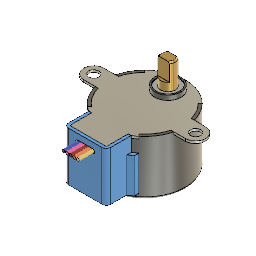
858 Stepper Motor 5VDC (Autodesk Fusion 360 design; units mm, degrees)
Autodesk Fusion 360 part; units mm, degrees
note: some values were not read from the file. Chosen so that the rebuilt part matches the saved one: which face or edge a step refers to.
sketch "base" plane through (0, 0, 0) normal (0, 0, 1) x (1, 0, 0)
  circle A0 centre (-17.5, 0) radius 1.75
  circle A1 centre (17.5, 0) radius 1.75
  line L0 (-17.5, 0) -> (17.5, 0) construction
  circle A2 centre (0, 0) radius 14
  line L1 (-21, 3.5) -> (21, 3.5)
  line L2 (21, 3.5) -> (21, -3.5)
  line L3 (21, -3.5) -> (-21, -3.5)
  line L4 (-21, -3.5) -> (-21, 3.5)
  line L5 (-7.3, -10.5) -> (7.3, -10.5)
  line L6 (7.3, -10.5) -> (7.3, -20.5)
  line L7 (7.3, -20.5) -> (-7.3, -20.5)
  line L8 (-7.3, -20.5) -> (-7.3, -10.5)
  line L9 (0, -10.5) -> (0, 0) construction
  circle A3 centre (0, 8) radius 4.5
  line L10 (0, 8) -> (0, 0) construction
  dimension "d1" = 3.5
  dimension "d2" = 3.5
  dimension "d5" = 7
  dimension "d6" = 3.5
  dimension "d7" = 3.5
  dimension "d9" = 3.5
  dimension "d10" = 28
  dimension "d12" = 10
  dimension "d14" = 17
  dimension "d15" = 14.6
  dimension "d16" = 9
  dimension "d17" = 8
  dimension "d56" = 35
  measures "d1" diameter of A0
  measures "d2" diameter of A1
  measures "d5" distance of L1.start L3.end
  measures "d6" distance of A2.centre L1
  measures "d7" distance of A1.centre L2
  measures "d9" distance of A0.centre L4
  measures "d10" diameter of A2
  measures "d12" distance of L5.start L7.end
  measures "d14" distance of L3 L7
  measures "d15" distance of L6.end L7.end
  measures "d16" diameter of A3
  measures "d17" distance of A2.centre A3.centre
  measures "d56" distance of A0.centre A1.centre
extrude "Extrude1" add sketch "base" against normal blind 0.8 contours A2 L1 L3 | A2 L1 L2 L3 | A3 | A2 L1 | A2 L3 L5 L6 L8 | A2 L1 L3 L4 | A2 L6 L7 L8 | A2 L5 L6 L8 makes body 1
fillet "Fillet1" radius 3.5 4 edges at (21, -3.5, -0.4) (21, 3.5, -0.4) (-21, 3.5, -0.4) (-21, -3.5, -0.4) on bodies 1
extrude "Extrude2" add sketch "base" against normal blind 19 contours A2 L1 L3 | A3 | A2 L1 | A2 L3 L5 L6 L8 | A2 L6 L7 L8 | A2 L5 L6 L8 bodies 1
extrude "Extrude3" add sketch "base" along normal blind 1.6 contours A3 bodies 1
sketch "coupler" plane through (0, 0, 1.6) normal (0, 0, 1) x (-1, 0, 0)
  circle A0 centre (0, -8) radius 4.5
  circle A1 centre (0, -8) radius 2.5
  circle A2 centre (0, -8) radius 4
  dimension "d25" = 5
  dimension "d62" = 0.5
  measures "d25" diameter of A1
extrude "Extrude14" cut sketch "coupler" against normal blind 1.6 contours A1 | A2 bodies 1
extrude "Extrude15" add sketch "coupler" against normal blind 1.6 separate body contours A1 | A2 makes body 2
extrude "Extrude4" add sketch "coupler" along normal blind 2.4 separate body contours A1 makes body 3
sketch "shaft" plane through (0, 0, 4) normal (0, 0, 1) x (-1, 0, 0)
  circle A0 centre (0, -8) radius 2.5
  circle A1 centre (0, -8) radius 2.5
  line L0 (2.5, -9.5) -> (-2.5, -9.5)
  line L1 (-2.5, -9.5) -> (-2.5, -6.5)
  line L2 (-2.5, -6.5) -> (2.5, -6.5)
  line L3 (2.5, -6.5) -> (2.5, -9.5)
  line L4 (0, -8) -> (0, -9.5) construction
  dimension "d28" = 5
  dimension "d31" = 3
  dimension "d32" = 5
  dimension "d33" = 1.5
  measures "d28" diameter of A1
  measures "d31" distance of L0.start L2.end
  measures "d32" distance of L0.start L0.end
  measures "d33" distance of A0.centre L4.end
extrude "Extrude5" add sketch "shaft" along normal blind 6 contours A0 A1 L0 L2 bodies 3
extrude "Extrude6" cut sketch "base" along normal blind 2 from surface at -19 contours A2 L6 L7 L8 bodies 1
fillet "Fillet2" radius 1.5 2 edges at (-7.3, -20.5, -8.5) (7.3, -20.5, -8.5) on bodies 1
fillet "Fillet3" radius 1 1 edges at (-13.0526, 5.0626, -19) on bodies 1
sketch "plate" plane through (0, 0, 0) normal (0, 0, 1) x (-1, 0, 0)
  arc A0 (-5.8, 20.5) -> (-7.3, 19) centre (-5.8, 19) ccw
  line L0 (-7.3, 19) -> (-7.3, 11.9461)
  arc A1 (-7.3, 11.9461) -> (-13.5554, 3.5) centre (0, 0) ccw
  line L1 (-13.5554, 3.5) -> (-17.5, 3.5)
  arc A2 (-17.5, 3.5) -> (-17.5, -3.5) centre (-17.5, 0) ccw
  line L2 (-17.5, -3.5) -> (-13.5554, -3.5)
  arc A3 (-13.5554, -3.5) -> (13.5554, -3.5) centre (0, 0) ccw
  line L3 (13.5554, -3.5) -> (17.5, -3.5)
  arc A4 (17.5, -3.5) -> (17.5, 3.5) centre (17.5, 0) ccw
  line L4 (17.5, 3.5) -> (13.5554, 3.5)
  arc A5 (13.5554, 3.5) -> (7.3, 11.9461) centre (0, 0) ccw
  line L5 (7.3, 11.9461) -> (7.3, 19)
  arc A6 (7.3, 19) -> (5.8, 20.5) centre (5.8, 19) ccw
  line L6 (5.8, 20.5) -> (-5.8, 20.5)
  circle A7 centre (0, -8) radius 4.5
  circle A8 centre (17.5, 0) radius 1.75
  circle A9 centre (-17.5, 0) radius 1.75
  line L7 (5.8, 19.5) -> (-5.8, 19.5)
  arc A10 (-5.8, 19.5) -> (-6.3, 19) centre (-5.8, 19) ccw
  line L8 (-6.3, 19) -> (-6.3, 11.3715)
  arc A11 (-6.3, 11.3715) -> (-12.7574, 2.5) centre (0, 0) ccw
  line L9 (-12.7574, 2.5) -> (-17.5, 2.5)
  arc A12 (-17.5, 2.5) -> (-17.5, -2.5) centre (-17.5, 0) ccw
  line L10 (-17.5, -2.5) -> (-12.7574, -2.5)
  arc A13 (-12.7574, -2.5) -> (12.7574, -2.5) centre (0, 0) ccw
  line L11 (12.7574, -2.5) -> (17.5, -2.5)
  arc A14 (17.5, -2.5) -> (17.5, 2.5) centre (17.5, 0) ccw
  line L12 (17.5, 2.5) -> (12.7574, 2.5)
  arc A15 (12.7574, 2.5) -> (6.3, 11.3715) centre (0, 0) ccw
  line L13 (6.3, 11.3715) -> (6.3, 19)
  arc A16 (6.3, 19) -> (5.8, 19.5) centre (5.8, 19) ccw
  line L14 (7.3, 11.9461) -> (-7.3, 11.9461)
  line L15 (13.5554, -3.5) -> (-13.5554, -3.5)
  line L16 (-13.5554, 3.5) -> (13.5554, 3.5)
  line L17 (10, 12) -> (5, 7)
  line L18 (5, 7) -> (-5, 7)
  line L19 (-5, 7) -> (-10, 12)
  line L20 (5, -5) -> (12.5, -12.5)
  line L21 (12.5, -12.5) -> (12.5, -15)
  line L22 (12.5, -15) -> (-12.5, -15)
  line L23 (-12.5, -15) -> (-12.5, -12.5)
  line L24 (-12.5, -12.5) -> (-5, -5)
  dimension "d39" = 1
extrude "Extrude7" cut sketch "plate" against normal up to surface (17 mm away) contours A0 L0 L5 A6 L6 L7 A10 L8 L13 A16 L14 bodies 1
extrude "Extrude8" add sketch "plate" against normal up to surface (17 mm away) separate body contours A0 L0 L5 A6 L6 L7 A10 L8 L13 A16 L14 makes body 4
chamfer "Chamfer1" distance 0.5 angle 45 3 edges at (-2.3717, 7.2094, 10) (2.5, 8, 10) (-2.3717, 8.7906, 10) on bodies 3
extrude "Extrude9" cut sketch "plate" against normal blind 0.8 contours A1 L8 A11 L14 L19 | L8 A11 A15 L13 L14 L17 L18 L19 | L7 A10 L8 L13 A16 L14 | A5 A15 L13 L14 L17 | L1 A2 L2 A11 L9 A12 L10 A13 L15 L16 | A11 A15 L16 L17 L18 L19 | A11 L9 A12 L10 A13 L11 A14 L12 A15 L15 L16 | L3 A4 L4 A13 L11 A14 L12 A15 L15 L16 | A3 A13 L20 L24 | A13 L15 bodies 1
extrude "Extrude11" add sketch "plate" against normal blind 0.8 separate body contours A1 L8 A11 L14 L19 | L8 A11 A15 L13 L14 L17 L18 L19 | L7 A10 L8 L13 A16 L14 | A5 A15 L13 L14 L17 | L1 A2 L2 A11 L9 A12 L10 A13 L15 L16 | A11 A15 L16 L17 L18 L19 | A11 L9 A12 L10 A13 L11 A14 L12 A15 L15 L16 | L3 A4 L4 A13 L11 A14 L12 A15 L15 L16 | A3 A13 L20 L24 | A13 L15 makes body 5
sketch "wire hole" plane through (0, -20.5, 0) normal (0, -1, 0) x (1, 0, 0)
  line L0 (-5.8, -17) -> (5.8, -17)
  line L1 (5.8, -17) -> (5.8, 0)
  line L2 (5.8, 0) -> (-5.8, 0)
  line L3 (-5.8, 0) -> (-5.8, -17)
  line L4 (-3.25, -2) -> (3.25, -2)
  line L5 (3.25, -2) -> (3.25, -3.5)
  line L6 (3.25, -3.5) -> (-3.25, -3.5)
  line L7 (-3.25, -3.5) -> (-3.25, -2)
  line L8 (0, -2) -> (0, 0) construction
  dimension "d51" = 2
  dimension "d52" = 6.5
  dimension "d61" = 1.5
  measures "d51" distance of L8.start L8.end
  measures "d52" distance of L5.end L6.end
  measures "d61" distance of L4.end L5.end
extrude "Extrude12" cut sketch "wire hole" against normal blind 1 contours L4 L5 L6 L7 bodies 4
fillet "Fillet4" radius 0.75 4 edges at (-3.25, -20, -3.5) (-3.25, -20, -2) (3.25, -20, -2) (3.25, -20, -3.5) on bodies 4
sketch "clip outline" plane through (0, 0, 0) normal (0, 0, 1) x (-1, 0, 0)
  arc A0 (7.3, 19) -> (5.8, 20.5) centre (5.8, 19) ccw
  line L0 (5.8, 20.5) -> (-5.8, 20.5)
  arc A1 (-5.8, 20.5) -> (-7.3, 19) centre (-5.8, 19) ccw
  line L1 (-7.3, 19) -> (-7.3, 11.9461)
  line L2 (-7.3, 11.9461) -> (-6.3, 11.9461)
  line L3 (-6.3, 11.9461) -> (-6.3, 19)
  arc A2 (-5.8, 19.5) -> (-6.3, 19) centre (-5.8, 19) ccw
  line L4 (-5.8, 19.5) -> (5.8, 19.5)
  arc A3 (6.3, 19) -> (5.8, 19.5) centre (5.8, 19) ccw
  line L5 (6.3, 19) -> (6.3, 11.9461)
  line L6 (6.3, 11.9461) -> (7.3, 11.9461)
  line L7 (7.3, 11.9461) -> (7.3, 19)
  line L8 (8.8489, 10.1647) -> (8.8489, 12.5)
  line L9 (8.8489, 12.5) -> (5.1772, 14.6198)
  circle A4 centre (0, -8) radius 4.5
  circle A5 centre (-17.5, 0) radius 1.75
  circle A6 centre (17.5, 0) radius 1.75
  arc A7 (-9.8995, -9.8995) -> (9.8995, -9.8995) centre (0, 0) ccw
  line L10 (9.8995, -9.8995) -> (9.1924, -9.1924)
  arc A8 (9.1924, -9.1924) -> (12.52, -3.5) centre (0, 0) ccw
  line L11 (12.52, -3.5) -> (17.5, -3.5)
  arc A9 (17.5, -3.5) -> (17.5, 3.5) centre (17.5, 0) ccw
  line L12 (17.5, 3.5) -> (12.52, 3.5)
  arc A10 (12.52, 3.5) -> (8.1378, 10.1378) centre (0, 0) ccw
  line L13 (8.1378, 10.1378) -> (8.8489, 10.8489)
  arc A11 (8.8489, 10.8489) -> (7.3, 11.9461) centre (0, 0) ccw
  line L14 (7.3, 11.9461) -> (6.3, 11.9461)
  line L15 (6.3, 11.9461) -> (6.3, 19)
  arc A12 (6.3, 19) -> (5.8, 19.5) centre (5.8, 19) ccw
  line L16 (5.8, 19.5) -> (-5.8, 19.5)
  arc A13 (-5.8, 19.5) -> (-6.3, 19) centre (-5.8, 19) ccw
  line L17 (-6.3, 19) -> (-6.3, 11.9461)
  line L18 (-6.3, 11.9461) -> (-7.3, 11.9461)
  arc A14 (-7.3, 11.9461) -> (-8.8489, 10.8489) centre (0, 0) ccw
  line L19 (-8.8489, 10.8489) -> (-8.1378, 10.1378)
  arc A15 (-8.1378, 10.1378) -> (-12.52, 3.5) centre (0, 0) ccw
  line L20 (-12.52, 3.5) -> (-17.5, 3.5)
  arc A16 (-17.5, 3.5) -> (-17.5, -3.5) centre (-17.5, 0) ccw
  line L21 (-17.5, -3.5) -> (-12.52, -3.5)
  arc A17 (-12.52, -3.5) -> (-9.1924, -9.1924) centre (0, 0) ccw
  line L22 (-9.1924, -9.1924) -> (-9.8995, -9.8995)
  line L23 (0, 19.5) -> (0, 12) construction
  line L24 (-8.8489, 10.1647) -> (-8.8489, 12.5)
  line L25 (-8.8489, 12.5) -> (-5.1772, 14.6198)
  dimension "d57" = 120
  measures "d57" angle of L8 L9
extrude "Extrude13" add sketch "clip outline" along normal blind 12 from surface at -17 contours L7 L8 L9 A11 | L1 A14 L24 L25 bodies 4
move_face "OffsetFaces1" offset -0.4 1 faces at (-1.2013, 8.5785, 1.6) on bodies 2
move_face "OffsetFaces2" offset 0.4 1 faces at (0.734, 7.4146, 1.6) on bodies 3
sketch "wires" plane through (0, -20.5, 0) normal (0, -1, 0) x (1, 0, 0)
  arc A0 (2.5, -3.5) -> (2.5, -2) centre (2.5, -2.75) ccw
  line L0 (2.5, -3.5) -> (-2.5, -3.5)
  arc A1 (-2.5, -2) -> (-2.5, -3.5) centre (-2.5, -2.75) ccw
  line L1 (-2.5, -2) -> (2.5, -2)
  line L2 (-5.8, -17) -> (5.8, -17)
  line L3 (5.8, -17) -> (5.8, 0)
  line L4 (5.8, 0) -> (-5.8, 0)
  line L5 (-5.8, 0) -> (-5.8, -17)
  circle A2 centre (-2.5, -2.75) radius 0.5
  circle A3 centre (-1.25, -2.75) radius 0.5
  circle A4 centre (0, -2.75) radius 0.5
  circle A5 centre (1.25, -2.75) radius 0.5
  circle A6 centre (2.5, -2.75) radius 0.5
  dimension "d69" = 1
  dimension "d72" = 1.25
  dimension "d73" = 0
  measures "d69" diameter of A2
extrude "Extrude16" add sketch "wires" along normal blind 6 from surface at -1 separate body contours A2 | A3 | A4 | A5 | A6 makes body 6 at (0.4994, -23.5, -2.7749) makes body 7 at (-0.7506, -23.5, -2.7749) makes body 8 at (1.7494, -23.5, -2.7749) makes body 9 at (-2.0006, -23.5, -2.7749) makes body 10 at (2.9994, -23.5, -2.7749)
equation "d6 = ( 7 / 2 ) * 1 mm"
equation "d20 = ( 7 / 2 ) * 1 mm"
equation "d55 = ( 1.5 / 2 ) * 1 mm"
named bodies: "motor body", "blue clip", "shalf rod", "top plate", "shaft coupler", "red", "pink", "orange", "blue", "yellow"
